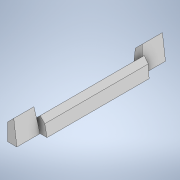
# Autodesk Inventor part: inside-join-2
Saved by Autodesk Inventor 2021 (Build 250183000, 183)
## iProperties
Created: 2020-12-08
Part Number: inside-join-2
Material: Generic
Document SubType Name: Modeling
Designer: Luke Kamols
Density: 1 g/cm^3
Appearance: Default
Author: Luke Kamols
Autodesk Inventor part; units mm, degrees
ref_plane "YZ Plane" through (0, 0, 0) normal (1, 0, 0) x (0, 1, 0)
ref_plane "XZ Plane" through (0, 0, 0) normal (0, 1, 0) x (-1, 0, 0)
ref_plane "XY Plane" through (0, 0, 0) normal (0, 0, 1) x (1, 0, 0)
sketch "Sketch1" plane through (0, 0, 0) normal (0, 0, 1) x (1, 0, 0)
  line L0 (0, 10) -> (3, 7)
  line L1 (0, 10) -> (4.2426, 10) construction
  line L2 (0, 10) -> (-4.2426, 10) construction
  line L3 (4.5, 0) -> (3, 7)
  line L4 (0, 0) -> (4.5, 0)
  line L5 (0, 10) -> (-3, 7)
  line L6 (0, 10) -> (-4.2426, 10) construction
  line L7 (-4.5, 0) -> (-3, 7)
  line L8 (0, 0) -> (-4.5, 0)
  dimension "d2" = 45
  constraints: 18 end point, 2 horizontal, 1 equal length
  measures "d2" angle of L0 L1
extrude "Extrusion1" add sketch "Sketch1" along normal blind 66
sketch "Sketch2" plane through (0, 0, 66) normal (0, 0, 1) x (1, 0, 0)
  line L0 (0, 0) -> (-6, 0)
  line L1 (-4.5, 0) -> (4.5, 0) projected
  line L2 (-6, 0) -> (-6, 11)
  line L3 (-6, 11) -> (-2, 15)
  line L4 (0, 0) -> (-2, 15)
  dimension "d8" = 6
  dimension "d9" = 11
  constraints: 8 end point, 1 collinear, 1 perpendicular
  measures "d8" distance of L0.start L0.end
  measures "d9" distance of L0.end L2.end
extrude "Extrusion2" add sketch "Sketch2" along normal blind 15
sketch "Sketch8" plane through (0, 0, 0) normal (0, 0, -1) x (-1, 0, 0)
  line L0 (1.1765, 8.8235) -> (3, 7) projected
  line L1 (3, 7) -> (4.5, 0) projected
  line L2 (6, 0) -> (4.5, 0) projected
  line L3 (6, 11) -> (6, 0) projected
  line L4 (2, 15) -> (6, 11) projected
  line L5 (1.1765, 8.8235) -> (2, 15) projected
  line L6 (0, 0) -> (2, 15) projected
  line L7 (2, 15) -> (6, 11) projected
  line L8 (6, 11) -> (6, 0) projected
  line L9 (6, 0) -> (0, 0) projected
extrude "Extrusion8" add sketch "Sketch8" along normal blind 15
sketch "Sketch13" plane through (0, 0, 81) normal (0.9912279, 0.1321637, 0) x (0, 0, -1)
  line L0 (15, 15.1327) -> (15, 11.6965) projected
  line L1 (15, 15.1327) -> (15, 0)
  line L2 (15, 15.1327) -> (13, 15.1327)
  line L3 (15, 15.1327) -> (0, 15.1327) projected
  line L4 (13, 15.1327) -> (15, 0)
  line L5 (15, 7.3351) -> (15, 0.5947) projected
  line L6 (15, 0.5947) -> (15, 0)
  line L7 (81, 15.1327) -> (96, 15.1327) projected
  line L8 (81, 15.1327) -> (81, 8.9016) projected
  line L9 (81, 0) -> (81, 8.9016) projected
  line L10 (81, 0) -> (96, 0) projected
  line L11 (15, 0) -> (0, 0) projected
  line L12 (15, 8.9016) -> (15, 0) projected
  line L13 (15, 8.9016) -> (15, 15.1327) projected
  line L14 (15, 15.1327) -> (0, 15.1327) projected
  line L15 (81, 15.1327) -> (81, 8.9016) projected
  line L16 (81, 15.1327) -> (83, 15.1327)
  line L17 (81, 15.1327) -> (94, 15.1327) projected
  line L18 (81, 0) -> (96, 0) projected
  line L19 (83, 15.1327) -> (81, 0)
  line L20 (0, 0) -> (0, 15.1327) projected
  line L21 (96, 15.1327) -> (96, 0) projected
  point P0 (2, 15.1327)
  dimension "d42" = 2
  dimension "d43" = 2
  constraints: 12 end point, 2 point on line, 1 collinear, 1 vertical
  measures "d42" distance of L0.start L2.end
  measures "d43" distance of L7.start L16.end
extrude "Extrusion11" cut sketch "Sketch13" against normal blind 12.225 contours L0 L1 L4 L2 | L7 L19 L9 L8
sketch "Sketch15" plane through (0, 0, 66) normal (0, 0, 1) x (1, 0, 0)
  line L0 (0, 0) -> (4.5, 0) projected
  line L1 (4.5, 0) -> (3, 7) projected
  line L2 (3, 7) -> (0, 10) projected
  line L3 (0, 10) -> (-3, 7) projected
  line L4 (-3, 7) -> (-4.5, 0) projected
  line L5 (0, 0) -> (-4.5, 0) projected
extrude "Extrusion12" add sketch "Sketch15" against normal up to surface surface through (-2, 15, -2) normal (0.0173167, -0.129875, -0.9913791)
body "Solid1"
